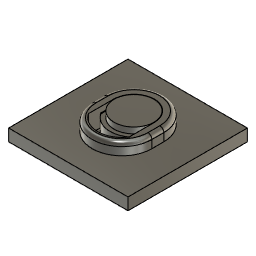
Subsurface Jaw Joint V3 (Autodesk Fusion 360 design; units mm, degrees)
Autodesk Fusion 360 part; units mm, degrees
sketch "Sketch1" plane through (0, 0, 0) normal (0, 0, 1) x (1, 0, 0)
  line L0 (-5, 1.5) -> (-5, -1.5)
  arc A0 (-5, -1.5) -> (5, -1.5) centre (0, -1.5) ccw
  line L1 (5, -1.5) -> (5, 1.5)
  arc A1 (5, 1.5) -> (-5, 1.5) centre (0, 1.5) ccw
  line L2 (0, 1.5) -> (0, -1.5) construction
  line L3 (-6, 1.5) -> (-6, -1.5)
  arc A2 (-6, -1.5) -> (6, -1.5) centre (0, -1.5) ccw
  line L4 (6, -1.5) -> (6, 1.5)
  arc A3 (6, 1.5) -> (-6, 1.5) centre (0, 1.5) ccw
  line L5 (0, 1.5) -> (0, -1.5) construction
  arc A4 (-5.1, -1.5) -> (5.1, -1.5) centre (0, -1.5) ccw
  line L6 (5.1, -1.5) -> (5.1, 1.5)
  arc A5 (5.1, 1.5) -> (-5.1, 1.5) centre (0, 1.5) ccw
  line L7 (-5.1, 1.5) -> (-5.1, -1.5)
  arc A6 (-6.1, -1.5) -> (6.1, -1.5) centre (0, -1.5) ccw
  line L8 (6.1, -1.5) -> (6.1, 1.5)
  arc A7 (6.1, 1.5) -> (-6.1, 1.5) centre (0, 1.5) ccw
  line L9 (-6.1, 1.5) -> (-6.1, -1.5)
  circle A8 centre (0, 1.5) radius 6.1
  circle A9 centre (0, 1.5) radius 6
  circle A10 centre (0, 1.5) radius 5
  line L10 (-5.1, 0) -> (-5.1, -8)
  line L11 (-5, 0) -> (-5, -8)
  line L12 (5, 0) -> (5, -8)
  line L13 (5.1, 0) -> (5.1, -8)
  arc A11 (7.5, 1.5) -> (-7.5, 1.5) centre (0, 1.5) ccw
  line L14 (-7.5, 1.5) -> (-7.5, -1.5)
  arc A12 (-7.5, -1.5) -> (7.5, -1.5) centre (0, -1.5) ccw
  line L15 (7.5, -1.5) -> (7.5, 1.5)
  line L16 (15, 15) -> (-15, 15)
  line L17 (-15, 15) -> (-15, -15)
  line L18 (-15, -15) -> (15, -15)
  line L19 (15, -15) -> (15, 15)
  line L20 (15, 15) -> (-15, -15) construction
  line L21 (-15, 15) -> (15, -15) construction
  line L22 (-5.1, 1.5) -> (-5.1, 9.5)
  line L23 (-5, 1.5) -> (-5, 9.5)
  line L24 (5, 1.5) -> (5, 9.5)
  line L25 (5.1, 1.5) -> (5.1, 9.5)
  dimension "d55" = 10
  dimension "d56" = 12
  dimension "d57" = 0.1
  dimension "d58" = 0.1
  dimension "d59" = 8
  dimension "d60" = 8
  dimension "d61" = 8
  dimension "d62" = 8
  dimension "d65" = 1.5
  dimension "d74" = 8
  constraint tangent L0 A0
  constraint tangent A0 L1
  constraint parallel L0 L1
  constraint tangent L1 A1
  constraint tangent L0 A1
  constraint vertical L2
  constraint tangent L3 A2
  constraint tangent A2 L4
  constraint parallel L3 L4
  constraint tangent L4 A3
  constraint tangent L3 A3
  constraint coincident A0.centre L2.end
  constraint parallel L2 L5
  constraint coincident A1.centre L2.start
  constraint concentric A3 A8
  constraint coincident A7.end A8
  constraint concentric A8 A9
  constraint coincident L3.start A9
  constraint tangent L3 A9
  constraint concentric A3 A10
  constraint coincident L0.start A10
  constraint vertical L10
  constraint midpoint L7 L10.start
  constraint vertical L11
  constraint midpoint L0 L11.start
  constraint vertical L12
  constraint midpoint L1 L12.start
  constraint vertical L13
  constraint midpoint L6 L13.start
  constraint horizontal L16
  constraint perpendicular L16 L17
  constraint parallel L16 L18
  constraint parallel L17 L19
  constraint coincident L20 origin
  constraint coincident L21 origin
  constraint vertical L22
  constraint tangent A1 L23
  constraint vertical L23
  constraint tangent A1 L24
  constraint vertical L24
  constraint tangent A5 L25
  constraint parallel L24 L25
  measures "d55" diameter of A0
  measures "d56" diameter of A2
  measures "d59" distance of L10.start L10.end
  measures "d60" distance of L11.start L11.end
  measures "d61" distance of L12.start L12.end
  measures "d62" distance of L13.start L13.end
  measures "d74" distance of A5.end L22.end
extrude "Extrude12" add sketch "Sketch1" against normal blind 1.4 contours L0 A0 L1 A9 A10 L11 L12 | A1 A5 A10 L23 L24 | A1 A10 | L0 A4 A5 L7 A9 L10 L11 L23 | L1 A4 L6 A5 A9 L12 L13 L24 | A3 A5 A9 L23 L24 | A3 A5 A9 L22 L23 | A0 A9 L11 | A3 A5 A9 L24 L25 | A3 A4 L7 A9 L10 L22 | A3 A7 A8 A9 L23 L24 | A3 A7 A8 A9 L22 L23 | A0 A8 A9 | A0 A8 A9 L11 | A4 A8 A9 L11 | A0 A9 L12 | A3 A4 L6 A9 L13 L25 | A3 A7 A8 A9 L24 L25 | L3 A3 A7 A8 A9 L22 | A7 A8 A11 L23 L24 | A7 A8 A11 L22 L23 | A0 A8 | A0 A4 A8 L11 L12 | A0 A8 A9 L12 | L3 A8 A9 L10 | A4 A8 L10 | A4 A8 L11 | A4 A8 A9 L12 | L4 A3 A7 A8 A9 L25 | A7 A8 A11 L24 L25 | A6 A7 L9 A8 L10 A11 L14 A12 L22 | A2 A4 A8 L10 L11 | L3 A2 A8 L10 | A2 A4 L11 L12 | A4 A8 L13 | L4 A8 A9 L13 | A4 A8 L12 | A6 L8 A7 A8 L13 A11 A12 L15 L25 | L3 A2 A6 L9 A8 L10 | A2 A6 L10 L11 | A2 A4 A8 L12 L13 | A2 A6 L11 L12 | A2 L4 A8 L13 | A2 L4 A6 L8 A8 L13 | A6 L10 L11 A12 | A2 A6 L12 L13 | A6 L11 L12 A12 | A6 L12 L13 A12 | L16 L17 L18 L19 makes body 1
extrude "Extrude13" add sketch "Sketch1" along normal blind 3.2 contours A7 A8 A11 L23 L24 | A7 A8 A11 L22 L23 | A7 A8 A11 L24 L25 | A6 A7 L9 A8 L10 A11 L14 A12 L22 | L3 A2 A8 L10 | A6 L8 A7 A8 L13 A11 A12 L15 L25 | L3 A2 A6 L9 A8 L10 | A2 L4 A8 L13 | A2 L4 A6 L8 A8 L13 | A6 L10 L11 A12 | A6 L11 L12 A12 | A6 L12 L13 A12 | L16 L17 L18 L19 bodies 1
extrude "Extrude14" add sketch "Sketch1" along normal blind 1.4 from surface at 3.2 contours A3 A5 A9 L23 L24 | A3 A5 A9 L22 L23 | A3 A5 A9 L24 L25 | A3 L7 A9 L10 L22 | A3 A7 A8 A9 L23 L24 | A3 A7 A8 A9 L22 L23 | A3 L6 A9 L13 L25 | A3 A7 A8 A9 L24 L25 | L3 A3 A7 A8 A9 L22 | A7 A8 A11 L23 L24 | A7 A8 A11 L22 L23 | L4 A3 A7 A8 A9 L25 | A7 A8 A11 L24 L25 | L3 A8 A9 L10 | A6 A7 L9 A8 L10 A11 L14 A12 L22 | L4 A8 A9 L13 | A6 L8 A7 A8 L13 A11 A12 L15 L25 | L3 A2 A8 L10 | L3 A2 A6 L9 A8 L10 | A2 L4 A6 L8 A8 L13 | A2 L4 A8 L13 | A6 L10 L11 A12 | A6 L11 L12 A12 | A6 L12 L13 A12 bodies 1
extrude "Extrude15" cut 1 faces at (-12.5, 0.5, 3.2) along direction (0, 0, -1) blind 1.6 on bodies 1 bodies 1
extrude "Extrude16" add sketch "Sketch1" along normal blind 3 from surface at 0.1 separate body contours L0 A0 L1 A9 A10 L11 L12 | A1 A5 A10 L23 L24 | A1 A10 | A3 A5 A9 L23 L24 makes body 2
extrude "Extrude17" add sketch "Sketch1" along normal blind 1.5 from surface at 3.1 contours A1 A10 bodies 2
fillet "Fillet4" radius 1 4 edges at (7.5, 0, 4.6) (0, 9, 4.6) (-7.5, 0, 4.6) (0, -9, 4.6) on bodies 1
